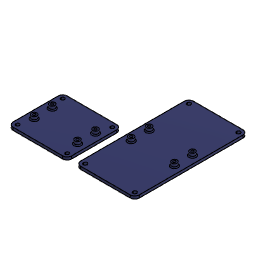
Lower Bay Tray - Creality MOSFET (Autodesk Fusion 360 design; units mm, degrees)
Autodesk Fusion 360 part; units mm, degrees
sketch "Sketch1" plane through (0, 0, 0) normal (0, 0, 1) x (1, 0, 0)
  line L0 (-65, 70) -> (-10, 70) construction
  line L1 (-10, 70) -> (-10, 20) construction
  line L2 (-10, 20) -> (-65, 20) construction
  line L3 (-65, 20) -> (-65, 70) construction
  line L4 (-70, 20) -> (-70, 70)
  arc A0 (-65, 75) -> (-70, 70) centre (-65, 70) ccw
  arc A1 (-5, 70) -> (-10, 75) centre (-10, 70) ccw
  line L5 (-5, 70) -> (-5, 20)
  line L6 (-65, 75) -> (-10, 75)
  arc A2 (-70, 20) -> (-65, 15) centre (-65, 20) ccw
  line L7 (-10, 15) -> (-65, 15)
  arc A3 (-10, 15) -> (-5, 20) centre (-10, 20) ccw
  line L8 (-66.8, 70.25) -> (-66.8, 69.75)
  arc A4 (-66.8, 69.75) -> (-63.2, 69.75) centre (-65, 69.75) ccw
  line L9 (-63.2, 69.75) -> (-63.2, 70.25)
  arc A5 (-63.2, 70.25) -> (-66.8, 70.25) centre (-65, 70.25) ccw
  line L10 (-65, 70.25) -> (-65, 69.75) construction
  line L11 (-37.5, 75) -> (-37.5, 15) construction
  line L12 (-70, 45) -> (-5, 45) construction
  arc A6 (-66.8, 19.75) -> (-63.2, 19.75) centre (-65, 19.75) ccw
  line L13 (-66.8, 19.75) -> (-66.8, 20.25)
  arc A7 (-63.2, 20.25) -> (-66.8, 20.25) centre (-65, 20.25) ccw
  line L14 (-63.2, 20.25) -> (-63.2, 19.75)
  arc A8 (-8.2, 70.25) -> (-11.8, 70.25) centre (-10, 70.25) ccw
  line L15 (-8.2, 70.25) -> (-8.2, 69.75)
  arc A9 (-11.8, 69.75) -> (-8.2, 69.75) centre (-10, 69.75) ccw
  line L16 (-11.8, 69.75) -> (-11.8, 70.25)
  line L17 (-11.8, 20.25) -> (-11.8, 19.75)
  arc A10 (-8.2, 20.25) -> (-11.8, 20.25) centre (-10, 20.25) ccw
  line L18 (-8.2, 19.75) -> (-8.2, 20.25)
  arc A11 (-11.8, 19.75) -> (-8.2, 19.75) centre (-10, 19.75) ccw
  line L19 (70, 140) -> (70, 15) construction
  line L20 (70, 15) -> (5, 15) construction
  line L21 (5, 140) -> (70, 140) construction
  line L22 (5, 15) -> (5, 140) construction
  line L23 (10, 135) -> (65, 135) construction
  line L24 (65, 135) -> (65, 20) construction
  line L25 (65, 20) -> (10, 20) construction
  line L26 (10, 20) -> (10, 135) construction
  line L27 (65, 15) -> (10, 15)
  line L28 (5, 20) -> (5, 135)
  line L29 (10, 140) -> (65, 140)
  line L30 (70, 135) -> (70, 20)
  arc A12 (10, 140) -> (5, 135) centre (10, 135) ccw
  arc A13 (70, 135) -> (65, 140) centre (65, 135) ccw
  arc A14 (5, 20) -> (10, 15) centre (10, 20) ccw
  arc A15 (65, 15) -> (70, 20) centre (65, 20) ccw
  line L31 (8.1, 135.25) -> (8.1, 134.75)
  arc A16 (8.1, 134.75) -> (11.9, 134.75) centre (10, 134.75) ccw
  line L32 (11.9, 134.75) -> (11.9, 135.25)
  arc A17 (11.9, 135.25) -> (8.1, 135.25) centre (10, 135.25) ccw
  line L33 (10, 135.25) -> (10, 134.75) construction
  line L34 (37.5, 140) -> (37.5, 15) construction
  line L35 (5, 77.5) -> (70, 77.5) construction
  arc A18 (63.1, 134.75) -> (66.9, 134.75) centre (65, 134.75) ccw
  line L36 (63.1, 134.75) -> (63.1, 135.25)
  arc A19 (66.9, 135.25) -> (63.1, 135.25) centre (65, 135.25) ccw
  line L37 (66.9, 135.25) -> (66.9, 134.75)
  line L38 (66.9, 19.75) -> (66.9, 20.25)
  arc A20 (63.1, 19.75) -> (66.9, 19.75) centre (65, 19.75) ccw
  line L39 (63.1, 20.25) -> (63.1, 19.75)
  arc A21 (66.9, 20.25) -> (63.1, 20.25) centre (65, 20.25) ccw
  arc A22 (8.1, 19.75) -> (11.9, 19.75) centre (10, 19.75) ccw
  line L40 (8.1, 19.75) -> (8.1, 20.25)
  line L41 (11.9, 20.25) -> (11.9, 19.75)
  arc A23 (11.9, 20.25) -> (8.1, 20.25) centre (10, 20.25) ccw
  point P0 (-65, 70)
  point P1 (10, 135)
  point P2 (65, 135)
  point P3 (10, 20)
  point P4 (65, 20)
  point P5 (10, 135)
  dimension "d1" = 3.6
  dimension "d5" = 3.8
  constraint tangent L8 A4
  constraint tangent A4 L9
  constraint parallel L8 L9
  constraint tangent L9 A5
  constraint tangent L8 A5
  constraint vertical L10
  constraint coincident P0 L0.start
  constraint midpoint L10 P0
  constraint midpoint L6 L11.start
  constraint midpoint L7 L11.end
  constraint midpoint L4 L12.start
  constraint midpoint L5 L12.end
  constraint symmetric L8.start L12 A6.start
  constraint symmetric L8.end L12 L13.end
  constraint symmetric A4.end L12 A7.start
  constraint symmetric L9.end L12 A6.end
  constraint symmetric A4 L12 A7
  constraint symmetric A5 L12 A6
  constraint symmetric L8.start L11 A8.start
  constraint symmetric L8.end L11 L15.end
  constraint symmetric A4.end L11 A9.start
  constraint symmetric L9.end L11 A8.end
  constraint symmetric A4 L11 A9
  constraint symmetric A5 L11 A8
  constraint symmetric L11 A6.end L17.end
  constraint symmetric L11 A6.start L18.start
  constraint symmetric L11 A6 A11
  constraint symmetric L11 L13.end A10.start
  constraint symmetric L11 A7.start L17.start
  constraint symmetric L11 A7 A10
  constraint horizontal L23
  constraint vertical L24
  constraint horizontal L25
  constraint vertical L26
  constraint coincident P4 L24.end
  constraint coincident P5 P1
  constraint coincident L21 L29.start
  constraint parallel L25 L27
  constraint parallel L26 L28
  constraint parallel L23 L29
  constraint parallel L24 L30
  constraint coincident L21 L29.end
  constraint coincident P2 L23.end
  constraint coincident L22 L28.start
  constraint coincident P3 L25.end
  constraint tangent L31 A16
  constraint tangent A16 L32
  constraint parallel L31 L32
  constraint tangent L32 A17
  constraint tangent L31 A17
  constraint vertical L33
  constraint midpoint L33 P5
  constraint midpoint L21 L34.start
  constraint midpoint L20 L34.end
  constraint midpoint L28 L35.start
  constraint midpoint L19 L35.end
  constraint symmetric L31.start L34 A19.start
  constraint symmetric L31.end L34 A18.end
  constraint symmetric A16.end L34 A18.start
  constraint symmetric L32.end L34 L36.end
  constraint symmetric A16 L34 A18
  constraint symmetric A17 L34 A19
  constraint symmetric L31.start L35 A22.start
  constraint symmetric L31.end L35 L40.end
  constraint symmetric A16.end L35 L41.start
  constraint symmetric L32.end L35 A22.end
  constraint symmetric A16 L35 A23
  constraint symmetric A17 L35 A22
  constraint symmetric L35 A18.end L38.end
  constraint symmetric L35 A18.start L39.start
  constraint symmetric L35 A18 A21
  constraint symmetric L35 L36.end A20.start
  constraint symmetric L35 A19.start L38.start
  constraint symmetric L35 A19 A20
  measures "d1" diameter of A4
  measures "d5" diameter of A16
extrude "Extrude1" add sketch "Sketch1" along normal blind 3 contours L4 A0 A1 L5 L6 A2 L7 A3 makes body 1 in component "Lower Bay Tray - Creality MOSFET - Small"
extrude "Extrude1'" add sketch "Sketch1" along normal blind 3 separate body contours L27 L28 L29 L30 A12 A13 A14 A15 makes body 2 in component "Lower Bay Tray - Creality MOSFET - Large"
ref_plane "WorkPlane1" through (0, 0, 3) normal (0, 0, 1) x (1, 0, 0)
sketch "Sketch2" plane through (0, 0, 3) normal (0, 0, 1) x (1, 0, 0)
  arc A0 (-66.8, 19.75) -> (-63.2, 19.75) centre (-65, 19.75) ccw
  line L0 (-66.8, 19.75) -> (-66.8, 20.25)
  arc A1 (-63.2, 20.25) -> (-66.8, 20.25) centre (-65, 20.25) ccw
  line L1 (-63.2, 20.25) -> (-63.2, 19.75)
  arc A2 (-8.2, 70.25) -> (-11.8, 70.25) centre (-10, 70.25) ccw
  line L2 (-8.2, 70.25) -> (-8.2, 69.75)
  arc A3 (-11.8, 69.75) -> (-8.2, 69.75) centre (-10, 69.75) ccw
  line L3 (-11.8, 69.75) -> (-11.8, 70.25)
  arc A4 (-63.2, 70.25) -> (-66.8, 70.25) centre (-65, 70.25) ccw
  line L4 (-63.2, 70.25) -> (-63.2, 69.75)
  arc A5 (-66.8, 69.75) -> (-63.2, 69.75) centre (-65, 69.75) ccw
  line L5 (-66.8, 69.75) -> (-66.8, 70.25)
  arc A6 (-11.8, 19.75) -> (-8.2, 19.75) centre (-10, 19.75) ccw
  line L6 (-11.8, 19.75) -> (-11.8, 20.25)
  arc A7 (-8.2, 20.25) -> (-11.8, 20.25) centre (-10, 20.25) ccw
  line L7 (-8.2, 20.25) -> (-8.2, 19.75)
  arc A8 (-70, 20) -> (-65, 15) centre (-65, 20) ccw
  line L8 (-65, 15) -> (-10, 15)
  arc A9 (-10, 15) -> (-5, 20) centre (-10, 20) ccw
  line L9 (-5, 20) -> (-5, 70)
  arc A10 (-5, 70) -> (-10, 75) centre (-10, 70) ccw
  line L10 (-10, 75) -> (-65, 75)
  arc A11 (-65, 75) -> (-70, 70) centre (-65, 70) ccw
  line L11 (-70, 70) -> (-70, 20)
  arc A12 (66.9, 20.25) -> (63.1, 20.25) centre (65, 20.25) ccw
  line L12 (66.9, 20.25) -> (66.9, 19.75)
  arc A13 (63.1, 19.75) -> (66.9, 19.75) centre (65, 19.75) ccw
  line L13 (63.1, 19.75) -> (63.1, 20.25)
  arc A14 (11.9, 135.25) -> (8.1, 135.25) centre (10, 135.25) ccw
  line L14 (11.9, 135.25) -> (11.9, 134.75)
  arc A15 (8.1, 134.75) -> (11.9, 134.75) centre (10, 134.75) ccw
  line L15 (8.1, 134.75) -> (8.1, 135.25)
  arc A16 (8.1, 19.75) -> (11.9, 19.75) centre (10, 19.75) ccw
  line L16 (8.1, 19.75) -> (8.1, 20.25)
  arc A17 (11.9, 20.25) -> (8.1, 20.25) centre (10, 20.25) ccw
  line L17 (11.9, 20.25) -> (11.9, 19.75)
  arc A18 (63.1, 134.75) -> (66.9, 134.75) centre (65, 134.75) ccw
  line L18 (63.1, 134.75) -> (63.1, 135.25)
  arc A19 (66.9, 135.25) -> (63.1, 135.25) centre (65, 135.25) ccw
  line L19 (66.9, 135.25) -> (66.9, 134.75)
  arc A20 (5, 20) -> (10, 15) centre (10, 20) ccw
  line L20 (10, 15) -> (65, 15)
  arc A21 (65, 15) -> (70, 20) centre (65, 20) ccw
  line L21 (70, 20) -> (70, 135)
  arc A22 (70, 135) -> (65, 140) centre (65, 135) ccw
  line L22 (65, 140) -> (10, 140)
  arc A23 (10, 140) -> (5, 135) centre (10, 135) ccw
  line L23 (5, 135) -> (5, 20)
  line L24 (-37.5, 75) -> (-37.5, 15) construction
  line L25 (-13.5, 55) -> (-61.5, 55) construction
  line L26 (-61.5, 55) -> (-61.5, 35) construction
  line L27 (-61.5, 35) -> (-13.5, 35) construction
  line L28 (-13.5, 35) -> (-13.5, 55) construction
  line L29 (-13.5, 55) -> (-61.5, 35) construction
  line L30 (-61.5, 55) -> (-13.5, 35) construction
  circle A24 centre (-61.5, 55) radius 1.4
  circle A25 centre (-61.5, 35) radius 1.4
  circle A26 centre (-13.5, 55) radius 1.4
  circle A27 centre (-13.5, 35) radius 1.4
  circle A28 centre (-61.5, 55) radius 3
  circle A29 centre (-13.5, 55) radius 3
  circle A30 centre (-61.5, 35) radius 3
  circle A31 centre (-13.5, 35) radius 3
  line L31 (5, 77.5) -> (70, 77.5) construction
  line L32 (61.5, 87.5) -> (13.5, 87.5) construction
  line L33 (13.5, 87.5) -> (61.5, 67.5) construction
  line L34 (61.5, 87.5) -> (13.5, 67.5) construction
  line L35 (61.5, 67.5) -> (61.5, 87.5) construction
  line L36 (13.5, 67.5) -> (61.5, 67.5) construction
  line L37 (13.5, 87.5) -> (13.5, 67.5) construction
  circle A32 centre (13.5, 87.5) radius 3
  circle A33 centre (13.5, 87.5) radius 1.4
  circle A34 centre (13.5, 67.5) radius 1.4
  circle A35 centre (13.5, 67.5) radius 3
  circle A36 centre (61.5, 67.5) radius 3
  circle A37 centre (61.5, 67.5) radius 1.4
  circle A38 centre (61.5, 87.5) radius 3
  circle A39 centre (61.5, 87.5) radius 1.4
  line L38 (37.5, 15) -> (37.5, 140)
  point P0 (-37.5, 45)
  dimension "d15" = 48
  dimension "d16" = 20
  dimension "d17" = 2.8
  dimension "d18" = 2.8
  dimension "d19" = 2.8
  dimension "d20" = 2.8
  dimension "d21" = 1.6
  dimension "d22" = 1.6
  dimension "d23" = 1.6
  dimension "d24" = 1.6
  dimension "d25" = 1.6
  dimension "d26" = 1.6
  dimension "d27" = 1.6
  dimension "d28" = 1.6
  dimension "d29" = 48
  dimension "d30" = 20
  dimension "d31" = 2.8
  dimension "d32" = 2.8
  dimension "d33" = 2.8
  dimension "d34" = 2.8
  constraint midpoint L10 L24.start
  constraint midpoint L8 L24.end
  constraint horizontal L25
  constraint perpendicular L25 L26
  constraint parallel L25 L27
  constraint parallel L26 L28
  constraint coincident L29 P0
  constraint coincident L30 P0
  constraint midpoint L24 P0
  constraint coincident L25.end L26.start
  constraint coincident L26.end L27.start
  constraint coincident L25.start L28.end
  constraint coincident L27.end L28.start
  constraint midpoint L23 L31.start
  constraint midpoint L21 L31.end
  constraint horizontal L32
  constraint perpendicular L32 L37
  constraint parallel L32 L36
  constraint parallel L35 L37
  constraint coincident L32.end L33.start
  constraint coincident L34.end L36.start
  constraint coincident L32.start L34.start
  constraint coincident L33.end L35.start
  constraint midpoint L20 L38.start
  constraint midpoint L22 L38.end
  constraint midpoint L33 L38
  measures "d15" distance of L26.end L27.end
  measures "d16" distance of L25.end L26.end
  measures "d17" diameter of A24
  measures "d18" diameter of A25
  measures "d19" diameter of A26
  measures "d20" diameter of A27
  measures "d29" distance of L34.end L33.end
  measures "d30" distance of L34.end L32.end
  measures "d31" diameter of A33
  measures "d32" diameter of A34
  measures "d33" diameter of A39
  measures "d34" diameter of A37
extrude "Extrude2" add sketch "Sketch2" along normal blind 4 contours A28 | A29 | A30 | A31 bodies 1 in component "Lower Bay Tray - Creality MOSFET - Small"
extrude "Extrude2'" add sketch "Sketch2" along normal blind 4 contours A32 | A35 | A36 | A38 bodies 2 in component "Lower Bay Tray - Creality MOSFET - Large"
fillet "Fillet1" radius 1 4 edges at (58.703, 68.5848, 3) (58.703, 88.5848, 3) (10.703, 88.5848, 3) (10.703, 68.5848, 3) on bodies 2 in component "Lower Bay Tray - Creality MOSFET - Large"
fillet "Fillet1'" radius 1 4 edges at (-16.297, 36.0848, 3) (-64.297, 56.0848, 3) (-64.297, 36.0848, 3) (-16.297, 56.0848, 3) on bodies 1 in component "Lower Bay Tray - Creality MOSFET - Small"
component "Lower Bay Tray - Creality MOSFET - Small" placed x (1, 0, 0) y (0, 1, 0) z (0, 0, 1) at (0, 0, 0)
component "Lower Bay Tray - Creality MOSFET - Large" placed x (1, 0, 0) y (0, 1, 0) z (0, 0, 1) at (0, 0, 0)
equation "large_m4 = 4.6 mm"
equation "small_m4 = 3.8 mm"
equation "large_m3 = 3.6 mm"
equation "small_m3 = 2.8 mm"
equation "d17 = small_m3"
equation "d18 = small_m3"
equation "d19 = small_m3"
equation "d20 = small_m3"
equation "d31 = small_m3"
equation "d32 = small_m3"
equation "d33 = small_m3"
equation "d34 = small_m3"
